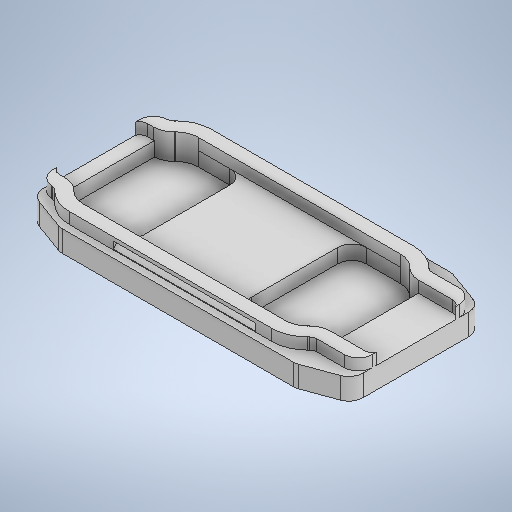
# Autodesk Inventor part: Housing_Lower
Saved by Autodesk Inventor 2025.1 (Build 291241020, 241B)
## iProperties
Created: 2024-09-09
Part Number: Housing_Lower
Material: Generic
Document SubType Name: Modeling
Designer: ahorat
Density: 1 g/cm^3
Appearance: Default
Author: ahorat
Autodesk Inventor part; units mm, degrees
ref_plane "YZ Plane" through (0, 0, 0) normal (1, 0, 0) x (0, 1, 0)
ref_plane "XZ Plane" through (0, 0, 0) normal (0, 1, 0) x (-1, 0, 0)
ref_plane "XY Plane" through (0, 0, 0) normal (0, 0, 1) x (1, 0, 0)
sketch "Sketch1" plane through (0, 0, 0) normal (0, 1, 0) x (-1, 0, 0)
  line L0 (-21.5822, -6.7784) -> (-16.7522, -6.7784)
  arc A0 (-14.5842, -7.6764) -> (-16.7522, -6.7784) centre (-16.751, -9.8416) ccw
  line L1 (-14.5842, -7.6764) -> (-14.4802, -7.7804)
  arc A1 (-14.4802, -7.7804) -> (-12.3122, -8.6784) centre (-12.3134, -5.6152) ccw
  line L2 (-12.3122, -8.6784) -> (16.1478, -8.6784)
  arc A2 (16.1478, -8.6784) -> (18.3158, -7.7804) centre (16.149, -5.6152) ccw
  line L3 (18.3158, -7.7804) -> (18.4198, -7.6764)
  arc A3 (20.5878, -6.7784) -> (18.4198, -7.6764) centre (20.5866, -9.8416) ccw
  line L4 (20.5878, -6.7784) -> (21.4178, -6.7784)
  arc A4 (21.4178, -6.7784) -> (22.4178, -5.7784) centre (21.4174, -5.778) ccw
  line L5 (22.4178, -5.7784) -> (22.4178, 4.4216)
  arc A5 (22.4178, 4.4216) -> (21.4178, 5.4216) centre (21.4174, 4.4213) ccw
  line L6 (21.4178, 5.4216) -> (20.5878, 5.4216)
  arc A6 (18.4198, 6.3196) -> (20.5878, 5.4216) centre (20.5866, 8.4848) ccw
  line L7 (18.4198, 6.3196) -> (18.3158, 6.4236)
  arc A7 (18.3158, 6.4236) -> (16.1478, 7.3216) centre (16.149, 4.2584) ccw
  line L8 (16.1478, 7.3216) -> (-12.3122, 7.3216)
  arc A8 (-12.3122, 7.3216) -> (-14.4802, 6.4236) centre (-12.3134, 4.2584) ccw
  line L9 (-14.4802, 6.4236) -> (-14.5842, 6.3196)
  arc A9 (-16.7522, 5.4216) -> (-14.5842, 6.3196) centre (-16.751, 8.4848) ccw
  line L10 (-16.7522, 5.4216) -> (-21.5822, 5.4216)
  arc A10 (-21.5822, 5.4216) -> (-22.5822, 4.4216) centre (-21.5819, 4.4213) ccw
  line L11 (-22.5822, 4.4216) -> (-22.5822, -5.7784)
  arc A11 (-22.5822, -5.7784) -> (-21.5822, -6.7784) centre (-21.5819, -5.778) ccw
  line L12 (19.8348, -9.0898) -> (19.7292, -9.1954)
  arc A12 (16.149, -10.6784) -> (19.7292, -9.1954) centre (16.149, -5.6152) ccw
  line L13 (16.149, -10.6784) -> (-12.3134, -10.6784)
  arc A13 (-15.8936, -9.1954) -> (-12.3134, -10.6784) centre (-12.3134, -5.6152) ccw
  line L14 (-15.8936, -9.1954) -> (-15.9992, -9.0898)
  arc A14 (-15.9992, -9.0898) -> (-16.751, -8.7784) centre (-16.751, -9.8416) ccw
  line L15 (-16.751, -8.7784) -> (-20.5822, -8.7784)
  line L16 (-20.5822, 7.4216) -> (-16.751, 7.4216)
  arc A15 (-16.751, 7.4216) -> (-15.9992, 7.733) centre (-16.751, 8.4848) ccw
  line L17 (-15.9992, 7.733) -> (-15.8936, 7.8387)
  arc A16 (-12.3134, 9.3216) -> (-15.8936, 7.8387) centre (-12.3134, 4.2584) ccw
  line L18 (-12.3134, 9.3216) -> (16.149, 9.3216)
  arc A17 (19.7292, 7.8387) -> (16.149, 9.3216) centre (16.149, 4.2584) ccw
  line L19 (19.7292, 7.8387) -> (19.8348, 7.733)
  arc A18 (19.8348, 7.733) -> (20.5866, 7.4216) centre (20.5866, 8.4848) ccw
  line L20 (20.5866, 7.4216) -> (20.4178, 7.4216)
  line L21 (20.4178, -8.7784) -> (20.5866, -8.7784)
  arc A19 (20.5866, -8.7784) -> (19.8348, -9.0898) centre (20.5866, -9.8416) ccw
  line L22 (22.4178, 5.4216) -> (22.4178, -6.7784)
  arc A20 (20.4178, -8.7784) -> (22.4178, -6.7784) centre (20.4178, -6.7784) ccw
  arc A21 (22.4178, 5.4216) -> (20.4178, 7.4216) centre (20.4178, 5.4216) ccw
  line L23 (-22.5822, 5.4216) -> (-22.5822, -6.7784)
  arc A22 (-22.5822, -6.7784) -> (-20.5822, -8.7784) centre (-20.5822, -6.7784) ccw
  arc A23 (-20.5822, 7.4216) -> (-22.5822, 5.4216) centre (-20.5822, 5.4216) ccw
  line L24 (16.149, -8.7784) -> (-12.3134, -8.7784)
  arc A24 (-14.5501, -7.8519) -> (-12.3134, -8.7784) centre (-12.3134, -5.6152) ccw
  line L25 (-14.5501, -7.8519) -> (-14.6557, -7.7463)
  arc A25 (-14.6557, -7.7463) -> (-16.751, -6.8784) centre (-16.751, -9.8416) ccw
  line L26 (-16.751, -6.8784) -> (-21.5819, -6.8784)
  arc A26 (-22.5822, -6.2363) -> (-21.5819, -6.8784) centre (-21.5819, -5.778) ccw
  arc A27 (-21.5819, 5.5216) -> (-22.5822, 4.8796) centre (-21.5819, 4.4213) ccw
  line L27 (-21.5819, 5.5216) -> (-16.751, 5.5216)
  arc A28 (-16.751, 5.5216) -> (-14.6557, 6.3895) centre (-16.751, 8.4848) ccw
  line L28 (-14.6557, 6.3895) -> (-14.5501, 6.4951)
  arc A29 (-12.3134, 7.4216) -> (-14.5501, 6.4951) centre (-12.3134, 4.2584) ccw
  line L29 (-12.3134, 7.4216) -> (16.149, 7.4216)
  arc A30 (18.3857, 6.4951) -> (16.149, 7.4216) centre (16.149, 4.2584) ccw
  line L30 (18.3857, 6.4951) -> (18.4913, 6.3895)
  arc A31 (18.4913, 6.3895) -> (20.5866, 5.5216) centre (20.5866, 8.4848) ccw
  line L31 (20.5866, 5.5216) -> (21.4174, 5.5216)
  arc A32 (22.4178, 4.8796) -> (21.4174, 5.5216) centre (21.4174, 4.4213) ccw
  arc A33 (21.4174, -6.8784) -> (22.4178, -6.2363) centre (21.4174, -5.778) ccw
  line L32 (21.4174, -6.8784) -> (20.5866, -6.8784)
  arc A34 (20.5866, -6.8784) -> (18.4913, -7.7463) centre (20.5866, -9.8416) ccw
  line L33 (18.4913, -7.7463) -> (18.3857, -7.8519)
  arc A35 (16.149, -8.7784) -> (18.3857, -7.8519) centre (16.149, -5.6152) ccw
  point P0 (-22.5822, -0.6784)
  point P1 (-22.5822, 4.4218)
  point P2 (22.4178, 4.4219)
  point P3 (22.4178, -5.7786)
  point P4 (-22.5822, -5.7785)
  dimension "d0" = 2
  dimension "d1" = 2
  dimension "d2" = 2
  dimension "d15" = 2
  dimension "d34" = 0.1
  constraints: 72 point on circle, 68 end point, 36 centre point, 8 tangent, 6 horizontal, 4 point on line, 4 vertical, 2 equal radius, 79 other
  measures "d0" radial gap between concentric circles of A3 A19
  measures "d1" radius of A20
  measures "d2" radius of A22
  measures "d15" distance between parallel lines of L18 L8
  measures "d34" distance between parallel lines of L2 L24
extrude "Extrusion1" add sketch "Sketch1" along normal blind 1.6 contours A26 L26 A25 L25 A24 L24 A35 L33 A34 L32 A33 L22 A20 L21 A19 L12 A12 L13 A13 L14 A14 L15 A22 L23 | L23 A23 L16 A15 L17 A16 L18 A17 L19 A18 L20 A21 L22 A32 L31 A31 L30 A30 L29 A29 L28 A28 L27 A27
sketch "Sketch2" plane through (0, 0, 0) normal (0, -1, 0) x (1, 0, 0)
  arc A0 (-22.4178, -6.7784) -> (-20.4178, -8.7784) centre (-20.4178, -6.7784) ccw projected
  line L0 (-22.4178, 4.8796) -> (-22.4178, -6.5074)
  line L1 (-20.4178, 7.4216) -> (-20.4178, -8.7784)
  arc A1 (22.5822, 5.4216) -> (20.5822, 7.4216) centre (20.5822, 5.4216) ccw projected
  arc A2 (20.5822, -8.7784) -> (22.5822, -6.7784) centre (20.5822, -6.7784) ccw projected
  line L2 (22.5822, 4.8796) -> (22.5822, -6.2363)
  line L3 (20.5822, -8.7784) -> (16.751, -8.7784) projected
  line L4 (16.751, 7.4216) -> (20.5822, 7.4216) projected
  line L5 (16.751, -8.7784) -> (16.751, 7.4216)
  line L6 (14.0619, 6.4196) -> (13.9579, 6.5236) construction
  arc A3 (13.9579, 6.5236) -> (11.7911, 7.4216) centre (11.7911, 4.3584) ccw construction
  line L7 (11.7911, 7.4216) -> (7.4843, 7.4216) construction
  line L8 (-18.6464, -8.3237) -> (-18.5319, -8.416) construction
  arc A4 (-18.5319, -8.416) -> (-17.9889, -8.7784) centre (-16.2569, -5.5955) ccw construction
  line L9 (-17.9889, -8.7784) -> (-11.6857, -8.7784) construction
  arc A5 (10.5359, -8.7784) -> (13.4025, -7.9533) centre (11.2292, -5.7946) ccw construction
  line L10 (13.4025, -7.9533) -> (13.5062, -7.849) construction
  circle A6 centre (12.1943, 5.3613) radius 1.15 construction
  circle A7 centre (7.4843, 0.5913) radius 0.5 construction
  circle A8 centre (9.4843, 0.5913) radius 0.5 construction
  circle A9 centre (9.4843, -1.9087) radius 0.5 construction
  circle A10 centre (12.1943, -6.6787) radius 1.15 construction
  circle A11 centre (7.4843, -1.9087) radius 0.5 construction
  circle A12 centre (-11.6857, -3.2087) radius 0.45 construction
  circle A13 centre (-11.6857, 0.8713) radius 0.45 construction
  circle A14 centre (-16.5257, 5.3413) radius 1.2 construction
  circle A15 centre (-14.2257, 1.8913) radius 0.45 construction
  circle A16 centre (-14.2257, -0.1487) radius 0.45 construction
  circle A17 centre (-11.6857, -1.1687) radius 0.45 construction
  circle A18 centre (-14.2257, -2.1887) radius 0.45 construction
  circle A19 centre (-16.5257, -6.6587) radius 1.2 construction
  line L11 (-9.6857, 5.4216) -> (-9.6857, -6.7784)
  line L12 (5.4843, -6.7784) -> (5.4843, 5.4216)
  arc A20 (7.4843, 7.4216) -> (5.4843, 5.4216) centre (7.4843, 5.4216) ccw
  arc A21 (-11.6857, -8.7784) -> (-9.6857, -6.7784) centre (-11.6857, -6.7784) ccw
  line L13 (7.4843, -8.7784) -> (6.6499, -8.7784)
  arc A22 (5.4843, -6.7784) -> (7.4843, -8.7784) centre (7.4843, -6.7784) ccw
  line L14 (-11.6857, 7.4216) -> (-12.246, 7.4216)
  arc A23 (-9.6857, 5.4216) -> (-11.6857, 7.4216) centre (-11.6857, 5.4216) ccw
  line L15 (-12.246, 7.4216) -> (7.4843, 7.4216)
  line L16 (12.3134, 7.4216) -> (-16.149, 7.4216) projected
  line L17 (-16.149, -8.7784) -> (12.3134, -8.7784) projected
  line L18 (-22.4178, -6.7784) -> (-22.4178, -6.2363) projected
  line L19 (16.751, -6.8784) -> (21.5819, -6.8784) projected
  arc A24 (21.5819, -6.8784) -> (22.5822, -6.2363) centre (21.5819, -5.778) ccw projected
  arc A25 (22.5822, 4.8796) -> (21.5819, 5.5216) centre (21.5819, 4.4213) ccw projected
  line L20 (21.5819, 5.5216) -> (16.751, 5.5216) projected
  line L21 (-20.5866, 5.5216) -> (-21.4174, 5.5216) projected
  arc A26 (-20.5866, 5.5216) -> (-18.4913, 6.3895) centre (-20.5866, 8.4848) ccw projected
  arc A27 (-21.4174, 5.5216) -> (-22.4178, 4.8796) centre (-21.4174, 4.4213) ccw projected
  line L22 (-21.4174, -6.8784) -> (-20.5866, -6.8784) projected
  arc A28 (-22.4178, -6.2363) -> (-21.4174, -6.8784) centre (-21.4174, -5.778) ccw projected
  arc A29 (-18.4913, -7.7463) -> (-20.5866, -6.8784) centre (-20.5866, -9.8416) ccw projected
  line L23 (22.5822, 5.4216) -> (22.5822, 4.8796) projected
  arc A30 (22.5822, 5.4216) -> (20.5822, 7.4216) centre (20.5822, 5.4216) ccw projected
  line L24 (16.751, 7.4216) -> (20.5822, 7.4216) projected
  arc A31 (15.9992, 7.733) -> (16.751, 7.4216) centre (16.751, 8.4848) ccw projected
  line L25 (15.8936, 7.8387) -> (15.9992, 7.733) projected
  arc A32 (15.8936, 7.8387) -> (12.3134, 9.3216) centre (12.3134, 4.2584) ccw projected
  line L26 (-16.149, 9.3216) -> (12.3134, 9.3216) projected
  arc A33 (-16.149, 9.3216) -> (-19.7292, 7.8387) centre (-16.149, 4.2584) ccw projected
  line L27 (-19.8348, 7.733) -> (-19.7292, 7.8387) projected
  arc A34 (-20.5866, 7.4216) -> (-19.8348, 7.733) centre (-20.5866, 8.4848) ccw projected
  line L28 (-20.4178, 7.4216) -> (-20.5866, 7.4216) projected
  arc A35 (-20.4178, 7.4216) -> (-22.4178, 5.4216) centre (-20.4178, 5.4216) ccw projected
  line L29 (-22.4178, 4.8796) -> (-22.4178, 5.4216) projected
  arc A36 (-21.4174, 5.5216) -> (-22.4178, 4.8796) centre (-21.4174, 4.4213) ccw projected
  line L30 (-20.5866, 5.5216) -> (-21.4174, 5.5216) projected
  arc A37 (-20.5866, 5.5216) -> (-18.4913, 6.3895) centre (-20.5866, 8.4848) ccw projected
  line L31 (-18.3857, 6.4951) -> (-18.4913, 6.3895) projected
  arc A38 (-16.149, 7.4216) -> (-18.3857, 6.4951) centre (-16.149, 4.2584) ccw projected
  line L32 (12.3134, 7.4216) -> (-16.149, 7.4216) projected
  arc A39 (14.5501, 6.4951) -> (12.3134, 7.4216) centre (12.3134, 4.2584) ccw projected
  line L33 (14.6557, 6.3895) -> (14.5501, 6.4951) projected
  arc A40 (14.6557, 6.3895) -> (16.751, 5.5216) centre (16.751, 8.4848) ccw projected
  line L34 (21.5819, 5.5216) -> (16.751, 5.5216) projected
  arc A41 (22.5822, 4.8796) -> (21.5819, 5.5216) centre (21.5819, 4.4213) ccw projected
  line L35 (20.5822, -8.7784) -> (16.751, -8.7784) projected
  arc A42 (20.5822, -8.7784) -> (22.5822, -6.7784) centre (20.5822, -6.7784) ccw projected
  line L36 (22.5822, -6.2363) -> (22.5822, -6.7784) projected
  arc A43 (21.5819, -6.8784) -> (22.5822, -6.2363) centre (21.5819, -5.778) ccw projected
  line L37 (16.751, -6.8784) -> (21.5819, -6.8784) projected
  arc A44 (16.751, -6.8784) -> (14.6557, -7.7463) centre (16.751, -9.8416) ccw projected
  line L38 (14.5501, -7.8519) -> (14.6557, -7.7463) projected
  arc A45 (12.3134, -8.7784) -> (14.5501, -7.8519) centre (12.3134, -5.6152) ccw projected
  line L39 (-16.149, -8.7784) -> (12.3134, -8.7784) projected
  arc A46 (-18.3857, -7.8519) -> (-16.149, -8.7784) centre (-16.149, -5.6152) ccw projected
  line L40 (-18.4913, -7.7463) -> (-18.3857, -7.8519) projected
  arc A47 (-18.4913, -7.7463) -> (-20.5866, -6.8784) centre (-20.5866, -9.8416) ccw projected
  line L41 (-21.4174, -6.8784) -> (-20.5866, -6.8784) projected
  arc A48 (-22.4178, -6.2363) -> (-21.4174, -6.8784) centre (-21.4174, -5.778) ccw projected
  line L42 (-22.4178, -6.7784) -> (-22.4178, -6.2363) projected
  arc A49 (-22.4178, -6.7784) -> (-20.4178, -8.7784) centre (-20.4178, -6.7784) ccw projected
  line L43 (-20.5866, -8.7784) -> (-20.4178, -8.7784) projected
  arc A50 (-19.8348, -9.0898) -> (-20.5866, -8.7784) centre (-20.5866, -9.8416) ccw projected
  line L44 (-19.7292, -9.1954) -> (-19.8348, -9.0898) projected
  arc A51 (-19.7292, -9.1954) -> (-16.149, -10.6784) centre (-16.149, -5.6152) ccw projected
  line L45 (12.3134, -10.6784) -> (-16.149, -10.6784) projected
  arc A52 (12.3134, -10.6784) -> (15.8936, -9.1954) centre (12.3134, -5.6152) ccw projected
  line L46 (15.9992, -9.0898) -> (15.8936, -9.1954) projected
  arc A53 (16.751, -8.7784) -> (15.9992, -9.0898) centre (16.751, -9.8416) ccw projected
  point P0 (0, 0)
  point P1 (-9.6857, 7.4216)
  point P2 (5.4843, -10.0483)
  point P3 (5.4843, 5.9259)
  point P4 (-2.3809, 7.4216)
  point P5 (-2.1007, -8.6784)
  point P6 (-20.4178, -6.8832)
  point P7 (-20.4178, 5.5264)
  point P8 (-18.4913, 6.3895)
  point P9 (22.5822, 4.8796)
  point P10 (22.5822, 5.4216)
  point P11 (-18.4913, -7.7463)
  point P12 (-20.4178, -8.7784)
  point P13 (22.5822, -6.2363)
  dimension "d6" = 2
  dimension "d7" = 2
  dimension "d8" = 2
  dimension "d9" = 2
  dimension "d10" = 2
  constraints: 28 end point, 21 centre point, 14 point on circle, 11 point on line, 10 tangent, 4 vertical, 3 coincident, 2 midpoint, 2 perpendicular, 1 equal radius, 1 parallel, 21 other
  measures "d6" distance from line of L11 A13.centre
  measures "d7" distance from line of L12 A7.centre
  measures "d8" radius of A20
  measures "d9" radius of A22
  measures "d10" radius of A23
extrude "Extrusion2" add sketch "Sketch2" along normal blind 2 contours L18 L0 A28 L22 A29 L1 A0 | L1 A29 L40 A46 L17 L13 A45 L38 A44 L5 A53 L46 A52 L45 A51 L44 A50 L43 | A29 L22 A28 L0 A27 L21 A26 L1 | A26 L21 A27 L29 A35 L1 | L1 L28 A34 L27 A33 L26 A32 L25 A31 L5 A40 L33 A39 L16 L15 L14 A38 L31 A26 | A21 L11 A23 L15 A20 L12 A22 L13 L17 | L5 L19 A24 L36 A2 L3 | L5 L20 A25 L2 A24 L19 | L5 L4 A1 L23 A25 L20
sketch "Sketch3" plane through (0, -2, 0) normal (0, -1, 0) x (1, 0, 0)
  arc A0 (-22.4178, -6.7784) -> (-20.4178, -8.7784) centre (-20.4178, -6.7784) ccw projected
  line L0 (-20.4178, -6.8832) -> (-20.4178, 5.5264) projected
  arc A1 (-20.4178, 5.5264) -> (-18.4913, 6.3895) centre (-20.5866, 8.4848) ccw projected
  line L1 (-20.4178, -8.7784) -> (-20.5866, -8.7784) projected
  arc A2 (-19.8348, -9.0898) -> (-20.5866, -8.7784) centre (-20.5866, -9.8416) ccw projected
  line L2 (-19.8348, -9.0898) -> (-19.7292, -9.1954) projected
  arc A3 (-19.7292, -9.1954) -> (-16.149, -10.6784) centre (-16.149, -5.6152) ccw projected
  line L3 (-16.149, -10.6784) -> (12.3134, -10.6784) projected
  arc A4 (12.3134, -10.6784) -> (15.8936, -9.1954) centre (12.3134, -5.6152) ccw projected
  line L4 (15.8936, -9.1954) -> (15.9992, -9.0898) projected
  arc A5 (16.751, -8.7784) -> (15.9992, -9.0898) centre (16.751, -9.8416) ccw projected
  line L5 (16.751, -8.7784) -> (20.5822, -8.7784) projected
  arc A6 (20.5822, -8.7784) -> (22.5822, -6.7784) centre (20.5822, -6.7784) ccw projected
  line L6 (22.5822, -6.7784) -> (22.5822, 5.4216) projected
  arc A7 (22.5822, 5.4216) -> (20.5822, 7.4216) centre (20.5822, 5.4216) ccw projected
  line L7 (20.5822, 7.4216) -> (16.751, 7.4216) projected
  arc A8 (15.9992, 7.733) -> (16.751, 7.4216) centre (16.751, 8.4848) ccw projected
  line L8 (15.9992, 7.733) -> (15.8936, 7.8387) projected
  arc A9 (15.8936, 7.8387) -> (12.3134, 9.3216) centre (12.3134, 4.2584) ccw projected
  line L9 (12.3134, 9.3216) -> (-16.149, 9.3216) projected
  arc A10 (-16.149, 9.3216) -> (-19.7292, 7.8387) centre (-16.149, 4.2584) ccw projected
  line L10 (-19.7292, 7.8387) -> (-19.8348, 7.733) projected
  arc A11 (-20.5866, 7.4216) -> (-19.8348, 7.733) centre (-20.5866, 8.4848) ccw projected
  line L11 (-20.5866, 7.4216) -> (-20.4178, 7.4216) projected
  arc A12 (-20.4178, 7.4216) -> (-22.4178, 5.4216) centre (-20.4178, 5.4216) ccw projected
  line L12 (-22.4178, 5.4216) -> (-22.4178, -6.7784) projected
  line L13 (-11.6857, -8.7784) -> (-16.149, -8.7784) projected
  arc A13 (-18.3857, -7.8519) -> (-16.149, -8.7784) centre (-16.149, -5.6152) ccw projected
  line L14 (-18.3857, -7.8519) -> (-18.4913, -7.7463) projected
  arc A14 (-18.4913, -7.7463) -> (-20.4178, -6.8832) centre (-20.5866, -9.8416) ccw projected
  line L15 (-18.4913, 6.3895) -> (-18.3857, 6.4951) projected
  arc A15 (-16.149, 7.4216) -> (-18.3857, 6.4951) centre (-16.149, 4.2584) ccw projected
  line L16 (-16.149, 7.4216) -> (-11.6857, 7.4216) projected
  arc A16 (-9.6857, 5.4216) -> (-11.6857, 7.4216) centre (-11.6857, 5.4216) ccw projected
  line L17 (-9.6857, 5.4216) -> (-9.6857, -6.7784) projected
  arc A17 (-11.6857, -8.7784) -> (-9.6857, -6.7784) centre (-11.6857, -6.7784) ccw projected
  point P0 (0, 0)
extrude "Extrusion3" add sketch "Sketch3" along normal blind 1 contours L12 A12 L11 A11 L10 A10 L9 A9 L8 A8 L7 A7 L6 A6 L5 A5 L4 A4 L3 A3 L2 A2 L1 A0 | L0 A1 L15 A15 L16 A16 L17 A17 L13 A13 L14 A14
sketch "Sketch4" plane through (0, -3, 0) normal (0, -1, 0) x (1, 0, 0)
  arc A0 (-22.4178, -6.7784) -> (-20.4178, -8.7784) centre (-20.4178, -6.7784) ccw projected
  line L0 (-16.149, 10.3216) -> (16.3134, 10.3216)
  line L1 (16.3134, -11.6784) -> (-16.149, -11.6784)
  line L2 (22.5822, -8.1246) -> (22.5822, 6.7679)
  line L3 (-22.4178, 5.4216) -> (-22.4178, -6.7784)
  arc A1 (21.2663, -10.004) -> (22.5822, -8.1246) centre (20.5822, -8.1246) ccw
  arc A2 (22.5822, 6.7679) -> (21.2663, 8.6473) centre (20.5822, 6.7679) ccw
  line L4 (-22.4178, -8.1246) -> (-22.4178, 6.7679)
  line L5 (-21.1018, 8.6473) -> (-16.833, 10.201)
  line L6 (-16.833, -11.5578) -> (-21.1018, -10.004)
  arc A3 (-21.1018, 8.6473) -> (-22.4178, 6.7679) centre (-20.4178, 6.7679) ccw
  arc A4 (-16.149, 10.3216) -> (-16.833, 10.201) centre (-16.149, 8.3216) ccw
  arc A5 (-16.833, -11.5578) -> (-16.149, -11.6784) centre (-16.149, -9.6784) ccw
  arc A6 (-22.4178, -8.1246) -> (-21.1018, -10.004) centre (-20.4178, -8.1246) ccw
  line L7 (16.9974, -11.5578) -> (21.2663, -10.004)
  line L8 (21.2663, 8.6473) -> (16.9974, 10.201)
  arc A7 (16.9974, 10.201) -> (16.3134, 10.3216) centre (16.3134, 8.3216) ccw
  arc A8 (16.3134, -11.6784) -> (16.9974, -11.5578) centre (16.3134, -9.6784) ccw
  arc A9 (-20.4178, 7.4216) -> (-22.4178, 5.4216) centre (-20.4178, 5.4216) ccw projected
  line L9 (-22.4178, 5.4216) -> (-22.4178, -6.7784) projected
  line L10 (-20.4178, -8.7784) -> (-20.5866, -8.7784) projected
  arc A10 (-19.8348, -9.0898) -> (-20.5866, -8.7784) centre (-20.5866, -9.8416) ccw projected
  line L11 (-19.8348, -9.0898) -> (-19.7292, -9.1954) projected
  arc A11 (-19.7292, -9.1954) -> (-16.149, -10.6784) centre (-16.149, -5.6152) ccw projected
  line L12 (-16.149, -10.6784) -> (12.3134, -10.6784) projected
  arc A12 (12.3134, -10.6784) -> (15.8936, -9.1954) centre (12.3134, -5.6152) ccw projected
  line L13 (15.8936, -9.1954) -> (15.9992, -9.0898) projected
  arc A13 (16.751, -8.7784) -> (15.9992, -9.0898) centre (16.751, -9.8416) ccw projected
  line L14 (16.751, -8.7784) -> (20.5822, -8.7784) projected
  arc A14 (20.5822, -8.7784) -> (22.5822, -6.7784) centre (20.5822, -6.7784) ccw projected
  line L15 (22.5822, -6.7784) -> (22.5822, 5.4216) projected
  arc A15 (22.5822, 5.4216) -> (20.5822, 7.4216) centre (20.5822, 5.4216) ccw projected
  line L16 (20.5822, 7.4216) -> (16.751, 7.4216) projected
  arc A16 (15.9992, 7.733) -> (16.751, 7.4216) centre (16.751, 8.4848) ccw projected
  line L17 (15.9992, 7.733) -> (15.8936, 7.8387) projected
  arc A17 (15.8936, 7.8387) -> (12.3134, 9.3216) centre (12.3134, 4.2584) ccw projected
  line L18 (12.3134, 9.3216) -> (-16.149, 9.3216) projected
  arc A18 (-16.149, 9.3216) -> (-19.7292, 7.8387) centre (-16.149, 4.2584) ccw projected
  line L19 (-19.7292, 7.8387) -> (-19.8348, 7.733) projected
  arc A19 (-20.5866, 7.4216) -> (-19.8348, 7.733) centre (-20.5866, 8.4848) ccw projected
  line L20 (-20.5866, 7.4216) -> (-20.4178, 7.4216) projected
  point P0 (0.0822, -11.6784)
  point P1 (22.5822, -0.6784)
  point P2 (-22.4178, -0.6784)
  point P3 (-22.4178, -6.7784)
  point P4 (22.5822, -6.7784)
  dimension "d16" = 2
  dimension "d19" = 2
  dimension "d20" = 4.2688
  dimension "d21" = 160
  dimension "d22" = 160
  dimension "d23" = 2
  constraints: 18 end point, 16 point on circle, 16 tangent, 8 centre point, 5 equal radius, 3 equal length, 3 midpoint, 3 vertical, 1 horizontal
  measures "d16" radius of A1
  measures "d19" radius of A3
  measures "d20" horizontal distance of L5.start L5.end
  measures "d21" angle of L0 L5
  measures "d22" angle of L8 L0
  measures "d23" radius of A7
extrude "Extrusion4" add sketch "Sketch4" against normal blind 3 contours A0 L10 A10 L11 A11 L12 A12 L13 A13 L14 A14 L2 A1 L7 A8 L1 A5 L6 A6 L4 | L4 A3 L5 A4 L0 A7 L8 A2 L2 A15 L16 A16 L17 A17 L18 A18 L19 A19 L20 A9
sketch "Sketch5" plane through (0, 0, 0) normal (1, 0, 0) x (0, 1, 0)
  line L0 (0, 9.3216) -> (1.6, 9.3216) projected
  line L1 (1.1, 9.3216) -> (0.6, 8.8216)
  line L2 (0.6, 8.8216) -> (0.1, 9.3216)
  line L3 (0, -10.6784) -> (1.6, -10.6784) projected
  line L4 (1.1, -10.6784) -> (0.6, -10.1784)
  line L5 (0.6, -10.1784) -> (0.1, -10.6784)
  point P0 (0, 0)
  dimension "d26" = 0.5
  dimension "d27" = 0.5
  dimension "d28" = 0.5
  dimension "d29" = 0.5
  constraints: 8 end point, 4 perpendicular, 4 point on line
  measures "d26" distance from line of L1.end L0
  measures "d27" distance of L0.end L1.start
  measures "d28" distance from line of L3 L4.end
  measures "d29" distance of L3.end L4.start
extrude "Extrusion5" cut sketch "Sketch5" along normal mid plane 20
body "Solid1"
